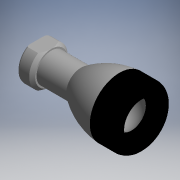
# Autodesk Inventor part: RBID6holder
Saved by Autodesk Inventor 2017.3 (Build 213256000, 256)
## iProperties
Part Number: RBID6holder
Material: Generic
Catalog Web Link: www.cadenas.de
Description: RBID, RBIDL-holder-Rod End Bearings - Link Ball Type with Thread - Link Ball Straight Type
Vendor: MISUMI
Document SubType Name: Modeling
Designer: partserver
Manufacturer: MISUMI
Mass: 4.99728 g
Surface Area: 28.4829 cm^2
Volume: 4.99728 cm^3
Density: 1 g/cm^3
Appearance: PSOLRGB-192-192-192
Category: PARTsolutions
Company: MISUMI
Title: RBID6holder
Author: Cadenas PARTsolutions
Comments: Rod End Bearings - Link Ball Type with Thread - Link Ball Straight Type
PSOL_IDENT_0: {$CADENAS_DATA\23d-libs\misumi\metric\34_cylinders\rbid_holder.prj},180 {VTYP=3D},{NB=RBID6holder},{
PSOL_IDENT_1: LINA=RBID6holder},{NN=RBID, RBIDL-holder},{DATE=30.06.2021 13:14:17},{GEOMDATE=04.07.2011 00:00:00},
PSOL_IDENT_2: {VERSION=},{LINEID=20},{WBVAR=TRS,MP},{WBNUMERIC=}  {NB=RBID6holder},{LINA=RBID6holder},{KT=DUMMY},{
PSOL_IDENT_3: PN=RBID6},{TYPE=RBID},{TRS=1},{TRS1='1', 'Right-Hand Thread', '2', 'Left-Hand Thread'},{MATH=High St
PSOL_IDENT_4: rength Zinc Alloy},{MATS=1035 Steel},{HARDS=20~28HRC},{MATB=NBR Type Special Synthetic Rubber},{HARD=
PSOL_IDENT_5: Sphere 650HV~},{M=6},{D=10.0},{D1=13},{D2=20},{L=55.2},{L1=28},{L2=15},{MP=1},{MPA='1','M6x1.0'},{L3=
PSOL_IDENT_6: 5.0},{W=11},{DD=6},{DDTOL=0/-0.030},{LL=27.2},{LL1=12.2},{LL2=11},{W1=8},{D3=10},{D4=20},{BD=12.700}
PSOL_IDENT_7: ,{ASF=25},{PK=3730},{SLCT=7450},{SLCC=14900},{MASS=40},{NDM=6},{P=1.00},{KDM=4.917},{PPATH=rbid_temp
PSOL_IDENT_8: l.prj},{RCS=0.03 or Less},{ACS=0.1 or Less}
NB: RBID6holder
NN: RBID, RBIDL-holder
NT: Rod End Bearings - Link Ball Type with Thread - Link Ball Straight Type
NBSYN: $PN.holder
LINA: RBID6holder
CATALOG: Misumi
PN: RBID6
TRS: Right-Hand Thread
MATH: High Strength Zinc Alloy
MATS: 1035 Steel
HARDS: 20~28HRC
MATB: NBR Type Special Synthetic Rubber
HARD: Sphere 650HV~
M: 6
D: 10
D1: 13
D2: 20
L: 55.2
L1: 28
L2: 15
MP: M6x1.0
L3: 5
W: 11
DD: 6
DDTOL: 0/-0.030
LL: 27.2
LL1: 12.2
LL2: 11
W1: 8
D3: 10
D4: 20
BD: 12.7
ASF: 25
PK: 3730
SLCT: 7450
SLCC: 14900
MASS: 40
PPATH: rbid_templ.prj
RCS: 0.03 or Less
ACS: 0.1 or Less
SUPPLIER: MISUMI
ARTICLENO: RBID6holder
BOMINFO: RBID6holder
CREATOR: CADENAS GmbH
Autodesk Inventor part; units mm, degrees
sketch "Sketch_1" plane through (0, 0, 0) normal (0, 0, 1) x (1, 0, 0)
  line L0 (28, 0) -> (-4.0667, 0)
  line L1 (13, 0) -> (13, 1.5)
  line L2 (13, 1.5) -> (6.1703, 1.5)
  arc A0 (6.1703, 1.5) -> (-4.0667, 4.877) centre (0, 0) ccw
  line L3 (-4.0667, 4.877) -> (-4.0667, 10)
  line L4 (-4.0667, 10) -> (0, 10)
  arc A1 (13, 5) -> (0, 10) centre (-2.0333, -14.6867) ccw
  line L5 (13, 5) -> (23, 5)
  line L6 (23, 5) -> (23, 5.5)
  line L7 (23, 5.5) -> (24, 6.5)
  line L8 (24, 6.5) -> (27.35, 6.5)
  arc A2 (28, 5.85) -> (27.35, 6.5) centre (27.35, 5.85) ccw
  line L9 (28, 5.85) -> (28, 0)
  line L10 (28, 0) -> (13, 0)
  constraints: 22 end point, 6 point on circle, 3 centre point
revolve "Revolution1" add sketch "Sketch_1" angle 360 about axis through (28, 0, 0) along (1, 0, 0)
sketch "Sketch_2" plane through (28, 0, 0) normal (1, 0, 0) x (0, 0, -1)
  line L0 (-22, 26) -> (-22, -26)
  line L1 (-22, -26) -> (22, -26)
  line L2 (22, -26) -> (22, 26)
  line L3 (22, 26) -> (-22, 26)
  line L4 (-5.5, 13) -> (-5.5, -13)
  line L5 (-5.5, -13) -> (5.5, -13)
  line L6 (5.5, -13) -> (5.5, 13)
  line L7 (5.5, 13) -> (-5.5, 13)
  constraints: 16 end point
extrude "Extrusion1" cut sketch "Sketch_2" against normal blind 5
sketch "Sketch_6" plane through (0, 0, 0) normal (0, 0, 1) x (1, 0, 0)
  line L0 (-2.0333, 0) -> (-8.1333, 0)
  arc A0 (-5.6933, 10) -> (-6.0214, 5.1422) centre (-5.6933, 7.56) ccw
  line L1 (-6.0214, 5.1422) -> (-4.0667, 4.877)
  arc A1 (-2.0333, 6.0157) -> (-4.0667, 4.877) centre (0, 0) ccw
  line L2 (-2.0333, 6.0157) -> (-2.0333, 10)
  line L3 (-2.0333, 10) -> (-5.6933, 10)
  constraints: 8 end point, 4 point on circle, 2 centre point
revolve "Revolution2" add sketch "Sketch_6" angle 360 about axis through (-2.0333, 0, 0) along (1, 0, 0)
sketch "Sketch4" plane through (28, -1.9931, -5.5) normal (1, 0, 0) x (0, 0, -1)
  point P0 (-5.5, 1.9931)
hole "Hole1" at (28, 0, 0) direction (-1, 0, 0) diameter 4.917 depth 16.5806 tip angle 120 countersink diameter 6 countersink angle 90 thread size "M6x1" class "6H" standard "ISO Metric profile"
ref_plane "holder_XY" through (0, 0, 0) normal (0, 0, 1) x (1, 0, 0)
ref_plane "holder_YZ" through (0, 0, 0) normal (1, 0, 0) x (0, 1, 0)
ref_plane "holder_ZX" through (0, 0, 0) normal (0, 1, 0) x (0, 0, 1)
body "Solid1"
